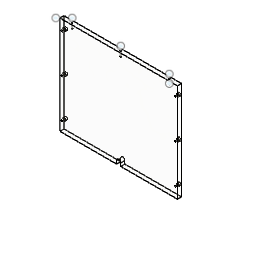
CAD_File 11 (Autodesk Fusion 360 design; units mm, degrees)
Autodesk Fusion 360 part; units mm, degrees
sketch "Sketch4" plane through (0, 107, 0) normal (0, 1, 0) x (-1, 0, 0)
  line L0 (-115, 0) -> (-107, 0)
  line L1 (-107, 0) -> (-107, 192)
  line L2 (-107, 192) -> (-115, 192)
  line L3 (-115, 192) -> (-115, 0)
  line L4 (-115, 192) -> (115, 192)
  line L5 (115, 192) -> (115, 0)
  line L6 (115, 0) -> (-115, 0)
  line L7 (-115, 0) -> (-115, 192)
  constraint horizontal L4
  constraint vertical L5
  constraint horizontal L6
  constraint vertical L7
  constraint coincident L2.end L3.start
extrude "Extrude10" add sketch "Sketch4" along normal blind 8
sketch "Sketch5" plane through (0, 115, 0) normal (0, 1, 0) x (-1, 0, 0)
  line L0 (-115, 0) -> (115, 0)
  line L1 (115, 0) -> (115, 192)
  line L2 (115, 192) -> (-115, 192)
  line L3 (-115, 192) -> (-115, 0)
  line L4 (0, 210) -> (0, -10) construction
  line L5 (130, 96) -> (-130, 96) construction
  circle A0 centre (-111, 172) radius 1.5
  circle A1 centre (-111, 96) radius 1.5
  circle A2 centre (-111, 172) radius 3
  circle A3 centre (-111, 96) radius 3
  circle A4 centre (111, 172) radius 1.5
  circle A5 centre (111, 172) radius 3
  circle A6 centre (111, 96) radius 1.5
  circle A7 centre (111, 96) radius 3
  circle A8 centre (-111, 20) radius 1.5
  circle A9 centre (-111, 20) radius 3
  circle A10 centre (111, 20) radius 3
  circle A11 centre (111, 20) radius 1.5
  dimension "d852" = 96
  dimension "d853" = 3
  dimension "d854" = 4
  dimension "d855" = 20
  dimension "d856" = 3
  dimension "d857" = 4
  dimension "d858" = 6
  dimension "d859" = 6
  constraint perpendicular L0 L4
  constraint perpendicular L1 L5
  constraint coincident L5 A1.centre
  constraint concentric A0 A2
  constraint concentric A1 A3
  constraint symmetric L4 A0 A4
  constraint symmetric L4 A1 A6
  constraint symmetric L4 A2 A5
  constraint symmetric L4 A3 A7
  constraint symmetric L5 A0 A8
  constraint symmetric L5 A2 A9
  constraint symmetric L5 A4 A11
  constraint symmetric L5 A5 A10
  measures "d852" distance of L2 L5
  measures "d853" diameter of A0
  measures "d854" distance of L3 A0.centre
  measures "d855" distance of L2 A0.centre
  measures "d856" diameter of A1
  measures "d857" distance of L3 A1.centre
  measures "d858" diameter of A2
  measures "d859" diameter of A3
extrude "Extrude11" cut sketch "Sketch5" against normal blind 18 contours A0 | A1 | A4 | A6 | A8 | A11
extrude "Extrude12" cut sketch "Sketch5" against normal blind 3 contours A2 | A3 | A5 | A7 | A9 | A10
sketch "sketch 1024" plane through (0, 0, 200) normal (0, 0, 1) x (-1, 0, 0)
  circle A0 centre (-95, -111) radius 1.5
  circle A1 centre (95, -111) radius 1.5
  circle A2 centre (111, -95) radius 1.5
  circle A3 centre (0, -111) radius 1.5
  circle A4 centre (-111, -95) radius 1.5
extrude "Extrude13" cut sketch "sketch 1024" against normal blind 18
thread "Thread1" "ISO Metric profile 3.0 M3x0.5 6H" major diameter 3.086 minor diameter 2.529 pitch 0.5 angle 60 resizes the face on face at (93.8043, 110.0943, 185.3333) on face at (-96.1957, 110.0943, 185.3333) on face at (-1.4536, 111.3701, 185.3333)
sketch "Sketch6" plane through (0, 115, 0) normal (0, 1, 0) x (-1, 0, 0)
  circle A0 centre (-111, 96) radius 3
  circle A1 centre (-111, 172) radius 3
  circle A2 centre (-111, 20) radius 3
  circle A3 centre (111, 96) radius 3
  circle A4 centre (111, 172) radius 3
  circle A5 centre (111, 20) radius 3
  line L0 (-115, 0) -> (115, 0)
  line L1 (115, 0) -> (115, 192)
  line L2 (115, 192) -> (-115, 192)
  line L3 (-115, 192) -> (-115, 0)
  line L4 (0, 0) -> (-4, 0)
  line L5 (-4, 0) -> (-4, 6)
  line L6 (0, 10) -> (0, 10)
  line L7 (4, 10) -> (4, 10.3244)
  line L8 (4, 6) -> (4, 0)
  arc A6 (0, 10) -> (-4, 6) centre (0, 6) ccw
  arc A7 (4, 6) -> (0, 10) centre (0, 6) ccw
  dimension "d934" = 4
  constraint coincident L4.start origin
  constraint coincident L0 L4.end
  constraint perpendicular L0 L5
  constraint perpendicular L0 L7
  constraint coincident L0 L8.end
  constraint perpendicular L0 L8
  constraint tangent L5 A6
  constraint coincident L7.start L6
  constraint coincident L7.end L8
  constraint tangent L8 A7
  constraint equal A6 A7
  measures "d934" radius of A6
extrude "Extrude14" cut sketch "Sketch6" against normal up to surface (8 mm away) contours L0 L4 L5 L8 A6 A7
